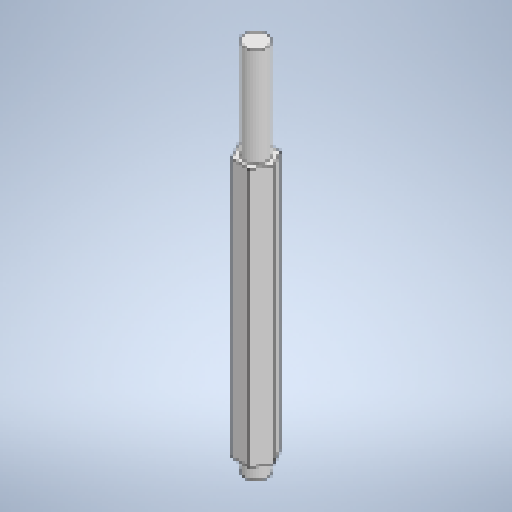
# Autodesk Inventor part: NVPH-201 shreder shaft
Saved by Autodesk Inventor 2025.1 (Build 291241020, 241B)
## iProperties
Created: 2024-12-04
Part Number: NVPH-201 shreder shaft
Material: Generic
Document SubType Name: Modeling
Designer: DELL
Density: 1 g/cm^3
Appearance: Default
Author: DELL
Autodesk Inventor part; units mm, degrees
ref_plane "YZ Plane" through (0, 0, 0) normal (1, 0, 0) x (0, 1, 0)
ref_plane "XZ Plane" through (0, 0, 0) normal (0, 1, 0) x (-1, 0, 0)
ref_plane "XY Plane" through (0, 0, 0) normal (0, 0, 1) x (1, 0, 0)
sketch "Sketch1" plane through (0, 0, 0) normal (0, 0, 1) x (1, 0, 0)
  line L0 (-11.547, -20) -> (-23.094, 0)
  line L1 (-23.094, 0) -> (-11.547, 20)
  line L2 (-11.547, 20) -> (11.547, 20)
  line L3 (11.547, 20) -> (23.094, 0)
  line L4 (23.094, 0) -> (11.547, -20)
  line L5 (11.547, -20) -> (-11.547, -20)
  point P0 (0, 0)
  point P1 (0, 0)
  dimension "d0" = 40
  constraints: 12 end point, 1 coincident, 1 horizontal, 13 other
  measures "d0" distance between parallel lines of L5 L2
extrude "Extrusion1" add sketch "Sketch1" along normal mid plane 340
sketch "Sketch2" plane through (0, 0, 0) normal (0, 0, 1) x (1, 0, 0)
  circle A0 centre (0, 0) radius 15
  dimension "d3" = 30
  constraints: 1 centre point, 1 coincident
  measures "d3" diameter of A0
extrude "Extrusion2" add sketch "Sketch2" along normal blind 300 and the other way blind 190
body "Solid1"
